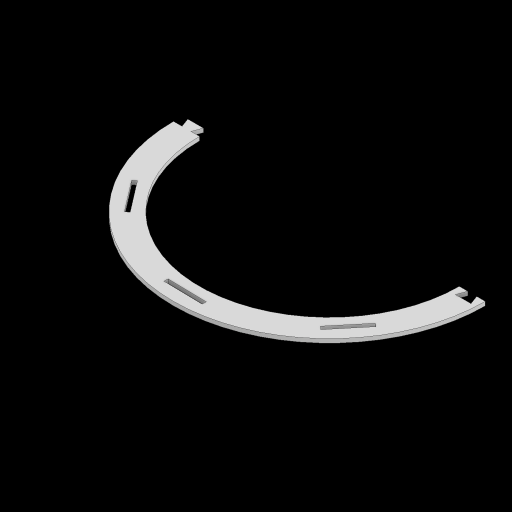
# Autodesk Inventor part: R7cm
Saved by Autodesk Inventor 2024.2 (Build 282272000, 272)
## iProperties
Created: 2024-10-01
Part Number: R7cm
Material: Generic
Document SubType Name: Modeling
Designer: jrcer
Density: 1 g/cm^3
Appearance: Default
Author: jrcer
Autodesk Inventor part; units mm, degrees
ref_plane "YZ Plane" through (0, 0, 0) normal (1, 0, 0) x (0, 1, 0)
ref_plane "XZ Plane" through (0, 0, 0) normal (0, 1, 0) x (-1, 0, 0)
ref_plane "XY Plane" through (0, 0, 0) normal (0, 0, 1) x (1, 0, 0)
sketch "Sketch1" plane through (0, 0, 0) normal (0, 1, 0) x (-1, 0, 0)
  circle A0 centre (0, 0) radius 100
  circle A1 centre (0, 0) radius 120
  line L0 (120, 0) -> (100, 0)
  line L1 (-120, 0) -> (-100, 0)
  line L2 (0, 0) -> (-100, 0) construction
  line L3 (0, 100) -> (0, 0) construction
  line L4 (0, 120) -> (0, 100)
  line L5 (-100, 0) -> (-120, 0)
  line L6 (-104, 7) -> (-116, 7)
  line L7 (-116, 7) -> (-113.4522, 0)
  line L8 (-104, 7) -> (-106.5478, 0)
  line L9 (-110, 0) -> (-110, 7) construction
  line L10 (-94.6848, 59.0429) -> (-75.5331, 82.1342)
  line L11 (-75.5331, 82.1342) -> (-73.07, 80.0914)
  line L12 (-73.07, 80.0914) -> (-92.2217, 57)
  line L13 (-92.2217, 57) -> (-94.6848, 59.0429)
  line L14 (-94.6848, 59.0429) -> (-73.07, 80.0914) construction
  line L15 (-75.5331, 82.1342) -> (-92.2217, 57) construction
  circle A2 centre (0, 0) radius 110 construction
  line L16 (104, -7) -> (106.5478, 0)
  line L17 (116, -7) -> (113.4522, 0)
  line L18 (104, -7) -> (116, -7)
  line L19 (-105.1966, -37.2149) -> (-111.3092, -7.8443)
  line L20 (-102.0637, -36.5629) -> (-105.1966, -37.2149)
  line L21 (-108.1763, -7.1923) -> (-102.0637, -36.5629)
  line L22 (-111.3092, -7.8443) -> (-108.1763, -7.1923)
  line L23 (-36.4932, -105.4491) -> (-63.2672, -91.9159)
  line L24 (-35.0496, -102.5932) -> (-36.4932, -105.4491)
  line L25 (-61.8237, -89.06) -> (-35.0496, -102.5932)
  line L26 (-63.2672, -91.9159) -> (-61.8237, -89.06)
  line L27 (59.6903, -94.278) -> (32.4162, -106.7729)
  line L28 (58.3575, -91.3687) -> (59.6903, -94.278)
  line L29 (31.0834, -103.8637) -> (58.3575, -91.3687)
  line L30 (32.4162, -106.7729) -> (31.0834, -103.8637)
  line L31 (110.9258, -12.1136) -> (103.6896, -41.2278)
  line L32 (107.8203, -11.3417) -> (110.9258, -12.1136)
  line L33 (100.5841, -40.4559) -> (107.8203, -11.3417)
  line L34 (103.6896, -41.2278) -> (100.5841, -40.4559)
  line L35 (78.6319, 79.1726) -> (96.8826, 55.3627)
  line L36 (76.0922, 77.2258) -> (78.6319, 79.1726)
  line L37 (94.3429, 53.416) -> (76.0922, 77.2258)
  line L38 (96.8826, 55.3627) -> (94.3429, 53.416)
  line L39 (-12.8735, 110.8402) -> (17.121, 110.264)
  line L40 (-12.9349, 107.6408) -> (-12.8735, 110.8402)
  line L41 (17.0596, 107.0646) -> (-12.9349, 107.6408)
  line L42 (17.121, 110.264) -> (17.0596, 107.0646)
  point P0 (110, 0)
  point P1 (-110, 0)
  point P2 (-83.8774, 69.5671)
  point P3 (-21.0302, 107.971)
  point P4 (-93.4533, 58.0214)
  point P5 (-74.3015, 81.1128)
  point P6 (110, -7)
  point P7 (-103.6301, -36.8889)
  point P8 (-109.7428, -7.5183)
  point P9 (-35.7714, -104.0212)
  point P10 (-62.5455, -90.4879)
  point P11 (59.0239, -92.8234)
  point P12 (31.7498, -105.3183)
  point P13 (109.373, -11.7276)
  point P14 (102.1369, -40.8419)
  point P15 (77.362, 78.1992)
  point P16 (95.6128, 54.3893)
  point P17 (-12.9042, 109.2405)
  point P18 (17.0903, 108.6643)
  point P19 (-106.5478, 0)
  point P20 (106.5478, 0)
  point P21 (113.4522, 0)
  dimension "d0" = 200
  dimension "d1" = 240
  dimension "d4" = 90
  dimension "d5" = 7
  dimension "d6" = 70
  dimension "d8" = 12
  dimension "d13" = 3.2
  dimension "d14" = 30
  dimension "d15" = 50
  dimension "d20" = 220
  dimension "d23" = 360
  dimension "d27" = 360
  constraints: 86 end point, 11 point on circle, 8 midpoint, 3 centre point, 3 coincident, 3 parallel, 2 horizontal, 2 horizontal alignment, 2 perpendicular, 2 point on line, 2 vertical, 1 collinear, 1 equal length, 88 other
  measures "d0" diameter of A0
  measures "d1" diameter of A1
  measures "d4" angle of L2 L3
  measures "d5" distance between parallel lines of L6 L5
  measures "d6" angle of L7 L6
  measures "d8" distance of L6.start L6.end
  measures "d13" distance of L10.end L11.end
  measures "d14" distance of L11.end L12.end
  measures "d15" vertical distance of L12.end L6.start
  measures "d20" diameter of A2
extrude "Extrusion1" add sketch "Sketch1" along normal blind 3 contours A0 L4 L41 L42 L39 A1 L0 | A0 L1 L8 L6 L7 A1 L4 L39 L40 L41 | L0 L17 L18 L16
body "Solid1"
